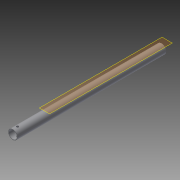
# Autodesk Inventor part: Launcher Crossbow
Saved by Autodesk Inventor 2014 SP1 (Build 180222100, 222)
## iProperties
Created: 2014-01-06
Part Number: Launcher Crossbow
Material: Generic
Document SubType Name: Modeling
Designer: Andrew Toennies
Density: 1 g/cm^3
Appearance: Default
Mass: 5.38384 g
Surface Area: 133.249 cm^2
Volume: 5.38384 cm^3
Author: Andrew Toennies
Autodesk Inventor part; units mm, degrees
ref_plane "YZ Plane" through (0, 0, 0) normal (1, 0, 0) x (0, 1, 0)
ref_plane "XY Plane" through (0, 0, 0) normal (0, 0, 1) x (1, 0, 0)
sketch "Sketch1" plane through (0, 0, 0) normal (0, 0, 1) x (1, 0, 0)
  circle A0 centre (0, 0) radius 6.35
  circle A1 centre (0, 0) radius 5.5372
  dimension "d0" = 12.7
  dimension "d1" = 11.0744
  constraints: 2 centre point, 2 coincident
  measures "d0" diameter of A0
  measures "d1" diameter of A1
extrude "Extrusion1" add sketch "Sketch1" along normal blind 177.8
ref_plane "Work Plane1" through (0, 6.35, 0) normal (0, 1, 0) x (-1, 0, 0)
sketch "Sketch2" plane through (0, 6.35, 0) normal (0, 1, 0) x (-1, 0, 0)
  circle A0 centre (0, 171.45) radius 1.5875
  line L0 (0, 171.45) -> (0, 0) construction
  dimension "d4" = 3.175
  dimension "d5" = 171.45
  constraints: 2 end point, 1 centre point, 1 vertical
  measures "d4" diameter of A0
  measures "d5" distance of L0.end L0.start
extrude "Extrusion2" cut sketch "Sketch2" against normal blind 25.4
body "Solid1"
